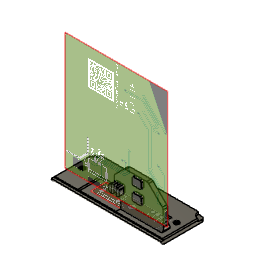
P3_LTE (Autodesk Fusion 360 design; units mm, degrees)
Autodesk Fusion 360 part; units mm, degrees
sketch "草图1" plane through (0, 0, 0) normal (0, 0, 1) x (1, 0, 0)
  line L0 (0, 0) -> (43, 0)
  line L1 (43, 0) -> (43, 17.2)
  line L2 (43, 17.2) -> (0, 17.2)
  line L3 (0, 17.2) -> (0, 0)
  line L4 (0, 17.2) -> (3, 17.2) construction
  line L5 (3, 17.2) -> (3, 9.2) construction
  line L6 (3, 9.2) -> (0, 9.2) construction
  line L7 (0, 9.2) -> (0, 17.2) construction
  line L8 (21.5, 17.2) -> (21.5, 0) construction
  circle A0 centre (3, 9.2) radius 1.025
  circle A1 centre (3, 9.2) radius 2.05
  circle A2 centre (40, 9.2) radius 1.025
  circle A3 centre (40, 9.2) radius 2.05
  dimension "d1" = 43
  dimension "d2" = 17.2
  dimension "d17" = 3
  dimension "d18" = 8
  dimension "d19" = 2.05
  dimension "d20" = 4.1
  constraint horizontal L0
  constraint vertical L1
  constraint horizontal L2
  constraint vertical L3
  constraint coincident L0.start L3.end
  constraint horizontal L4
  constraint vertical L5
  constraint horizontal L6
  constraint vertical L7
  constraint midpoint L2 L8.start
  constraint midpoint L0 L8.end
  constraint coincident L5.end L6.start
  constraint concentric A0 A1
  constraint symmetric L8 A0 A2
  constraint symmetric L8 A1 A3
  measures "d1" distance of L0.start L0.end
  measures "d2" distance of L0.start L2.end
  measures "d17" distance of L2.end L4.end
  measures "d18" distance of L2.end L6.end
  measures "d19" diameter of A0
  measures "d20" diameter of A1
extrude "拉伸1" add sketch "草图1" along normal blind 1.8 contours L0 L1 L2 L3 | A0 | A1 | A2 | A3
sketch "草图2" plane through (0, 0, 1.8) normal (0, 0, 1) x (-1, 0, 0)
  line L0 (0, -17.2) -> (0, 0)
  line L1 (0, 0) -> (-43, 0)
  line L2 (-43, 0) -> (-43, -17.2)
  line L3 (-43, -17.2) -> (0, -17.2)
  circle A0 centre (0, -17.2) radius 2.5
  circle A1 centre (-43, -17.2) radius 2.5
  line L4 (0, 0) -> (-43, 0)
  line L5 (-43, 0) -> (-43, -1)
  line L6 (-43, -1) -> (0, -1)
  line L7 (0, -1) -> (0, 0)
  dimension "d5" = 5
  dimension "d6" = 5
  dimension "d11" = 1
  constraint coincident L0.start L3.end
  constraint coincident L2.end L3.start
  constraint horizontal L4
  constraint vertical L5
  constraint horizontal L6
  constraint vertical L7
  constraint coincident L0.end L1.start
  measures "d5" diameter of A0
  measures "d6" diameter of A1
  measures "d11" distance of L0.end L6.end
extrude "拉伸2" cut sketch "草图2" against normal blind 0.9 contours L0 L3 A0 | L2 L3 A1 picked at (-1.3308, -16.2037) picked at (-41.5409, -16.4033)
fillet "圆角1" radius 1 2 edges at (43, 17.2, 0.45) (0, 17.2, 0.45)
extrude "拉伸3" cut sketch "草图2" against normal blind 0.4 contours L0 L1 L2 L4 L5 L6 L7
fillet "圆角3" radius 1.5 1 edges at (21.5, 0, 0)
chamfer "倒角1" distance 0.4 angle 45 2 edges at (43, 7.85, 1.8) (0, 7.85, 1.8)
extrude "拉伸4" cut sketch "草图1" along normal up to surface (1.8 mm away) contours A0 | A2
extrude "拉伸5" cut sketch "草图1" along normal blind 0.5 contours A1 | A3
chamfer "倒角3" distance 1 angle 45 2 edges at (39.0444, 9.5707, 0.5) (2.0444, 9.5707, 0.5)
chamfer "倒角4" distance 0.2 angle 45 2 edges at (1.0887, 8.4587, 0) (38.0887, 8.4587, 0)
sketch "草图10" plane through (0, 0, 1.8) normal (0, 0, 1) x (-1, 0, 0)
  circle A0 centre (-40, -9.2) radius 1.025
  circle A1 centre (-3, -9.2) radius 1.025
  line L0 (-0.4, -14.7322) -> (-0.4, -1)
  line L1 (-0.4, -1) -> (-42.6, -1)
  line L2 (-42.6, -1) -> (-42.6, -14.7322)
  arc A2 (-40.5, -17.2) -> (-42.6, -14.7322) centre (-43, -17.2) ccw
  line L3 (-40.5, -17.2) -> (-2.5, -17.2)
  arc A3 (-0.4, -14.7322) -> (-2.5, -17.2) centre (0, -17.2) ccw
  line L4 (-40, -9.2) -> (-37.3, -9.2) construction
  line L5 (-37.3, -10) -> (-9.3, -10)
  line L6 (-9.3, -10) -> (-9.3, -3.9)
  line L7 (-9.3, -3.9) -> (-37.3, -3.9)
  line L8 (-37.3, -3.9) -> (-37.3, -10)
  line L9 (-37.3, -9.2) -> (-37.3, -10) construction
  line L10 (-4, -16) -> (-39, -16) construction
  line L11 (-39, -16) -> (-39, -10) construction
  line L12 (-39, -10) -> (-4, -10)
  line L13 (-4, -10) -> (-4, -16) construction
  line L14 (-21.5, -16) -> (-21.5, -10) construction
  line L15 (-21.5, -17.2) -> (-21.5, -1) construction
  line L16 (-37.3, -10) -> (-25.1, -10) construction
  line L17 (-25.1, -10) -> (-25.1, -6.6) construction
  line L18 (-25.1, -6.6) -> (-37.3, -6.6) construction
  line L19 (-37.3, -6.6) -> (-37.3, -10) construction
  circle A4 centre (-25.1, -6.6) radius 0.9
  line L20 (-9.3, -3.9) -> (-24.3, -3.9)
  line L21 (-24.3, -3.9) -> (-24.3, -1.9)
  line L22 (-24.3, -1.9) -> (-9.3, -1.9)
  line L23 (-9.3, -1.9) -> (-9.3, -3.9)
  line L24 (0, -14.7) -> (0, -1)
  line L25 (-43, -1) -> (-43, -14.7)
  line L26 (0, -1) -> (-43, -1) construction
  line L27 (-43, -1) -> (-43, -2.4) construction
  line L28 (-43, -2.4) -> (0, -2.4) construction
  line L29 (0, -2.4) -> (0, -1) construction
  line L30 (0, -2.4) -> (-2.8, -2.4) construction
  line L31 (-43, -2.4) -> (-40.2, -2.4) construction
  line L32 (-2.8, -2.4) -> (-40.2, -2.4)
  line L33 (-40.2, -2.4) -> (-40.2, -3.8)
  line L34 (-40.2, -3.8) -> (-2.8, -3.8)
  line L35 (-2.8, -3.8) -> (-2.8, -2.4)
  line L36 (0, -1) -> (-2.4, -1) construction
  line L37 (-2.4, -1) -> (-2.4, -5.5) construction
  line L38 (-2.4, -5.5) -> (0, -5.5) construction
  line L39 (0, -5.5) -> (0, -1) construction
  line L40 (-43, -1) -> (-40.6, -1) construction
  line L41 (-40.6, -1) -> (-40.6, -5.5) construction
  line L42 (-40.6, -5.5) -> (-43, -5.5) construction
  line L43 (-43, -5.5) -> (-43, -1) construction
  line L44 (-2.4, -5.5) -> (-40.6, -5.5)
  line L45 (-40.6, -5.5) -> (-40.6, -1)
  line L46 (-40.6, -1) -> (-2.4, -1)
  line L47 (-2.4, -1) -> (-2.4, -5.5)
  line L48 (-2.4, -3.8) -> (-2.8, -3.8)
  line L49 (-2.4, -2.4) -> (-2.8, -2.4)
  line L50 (-40.2, -3.8) -> (-40.6, -3.8)
  line L51 (-40.6, -2.4) -> (-40.2, -2.4)
  line L52 (-37.3, -3.9) -> (-37.3, -3.8)
  dimension "d180" = 2.7
  dimension "d181" = 28
  dimension "d182" = 6.1
  dimension "d183" = 0.8
  dimension "d184" = 35
  dimension "d185" = 6
  dimension "d186" = 12.2
  dimension "d187" = 3.4
  dimension "d188" = 1.8
  dimension "d189" = 15
  dimension "d190" = 2
  dimension "d204" = 1.4
  dimension "d205" = 2.8
  dimension "d206" = 2.8
  dimension "d207" = 1.4
  dimension "d210" = 2.4
  dimension "d211" = 4.5
  dimension "d212" = 2.4
  dimension "d213" = 4.5
  constraint coincident A0.centre L4.start
  constraint horizontal L4
  constraint horizontal L5
  constraint vertical L6
  constraint horizontal L7
  constraint vertical L8
  constraint coincident L4.end L8
  constraint perpendicular L4 L9
  constraint horizontal L10
  constraint vertical L11
  constraint horizontal L12
  constraint vertical L13
  constraint collinear L5 L12
  constraint midpoint L10 L14.start
  constraint midpoint L12 L14.end
  constraint midpoint L3 L15.start
  constraint midpoint L1 L15.end
  constraint collinear L14 L15
  constraint horizontal L16
  constraint vertical L17
  constraint horizontal L18
  constraint vertical L19
  constraint coincident L17.end L18.start
  constraint horizontal L20
  constraint vertical L21
  constraint horizontal L22
  constraint vertical L23
  constraint horizontal L26
  constraint vertical L27
  constraint horizontal L28
  constraint vertical L29
  constraint coincident L24.end L26.start
  constraint perpendicular L24 L30
  constraint perpendicular L2 L31
  constraint horizontal L32
  constraint vertical L33
  constraint horizontal L34
  constraint vertical L35
  constraint horizontal L36
  constraint vertical L37
  constraint horizontal L38
  constraint vertical L39
  constraint horizontal L40
  constraint vertical L41
  constraint horizontal L42
  constraint vertical L43
  constraint coincident L25.start L26.end
  constraint horizontal L44
  constraint vertical L45
  constraint horizontal L46
  constraint vertical L47
  constraint coincident L47 L48.start
  constraint perpendicular L35 L48
  constraint coincident L30 L49.start
  constraint coincident L37 L49.start
  constraint coincident L45 L50.end
  constraint perpendicular L45 L50
  constraint coincident L45 L51.start
  constraint coincident L31 L51.start
  constraint coincident L34 L52.end
  constraint perpendicular L34 L52
  measures "d180" distance of A0.centre L4.end
  measures "d181" distance of L5.start L5.end
  measures "d182" distance of L5.start L7.end
  measures "d183" distance of L4.end L5.start
  measures "d184" distance of L10.start L10.end
  measures "d185" distance of L10.start L12.end
  measures "d186" distance of L5.start L16.end
  measures "d187" distance of L5.start L18.end
  measures "d188" diameter of A4
  measures "d189" distance of L6.end L20.end
  measures "d190" distance of L6.end L22.end
  measures "d204" distance of L24.end L28.end
  measures "d205" distance of L28.end L30.end
  measures "d206" distance of L27.end L31.end
  measures "d207" distance of L30.end L34.end
  measures "d210" distance of L24.end L36.end
  measures "d211" distance of L24.end L38.end
  measures "d212" distance of L25.start L40.end
  measures "d213" distance of L25.start L42.end
extrude "拉伸25" cut sketch "草图10" against normal blind 0.8 contours L21 L22 L23 L32 | L21 L23 L32 L34 | L7 L20 L21 L23 L34
extrude "拉伸24" cut sketch "草图10" against normal blind 0.8 contours L6 L7 L8 L20 L44 | L5 L6 L8 L12 L44
chamfer "倒角12" distance 0.8 angle 45 1 edges at (16.8, 1.9, 1.8)
sketch "草图12" plane through (0, 0, 1.8) normal (0, 0, 1) x (-1, 0, 0)
  line L0 (-9.3, -1.1) -> (-9.3, -10)
  line L1 (-9.3, -10) -> (-37.3, -10)
  line L2 (-37.3, -10) -> (-37.3, -3.9)
  line L3 (-37.3, -3.9) -> (-24.3, -3.9)
  line L4 (-24.3, -3.9) -> (-24.3, -1.1)
  line L5 (-24.3, -1.1) -> (-9.3, -1.1)
  line L6 (-0.4, -14.7322) -> (-0.4, -1)
  line L7 (-0.4, -1) -> (-42.6, -1)
  line L8 (-42.6, -1) -> (-42.6, -14.7322)
  arc A0 (-40.5, -17.2) -> (-42.6, -14.7322) centre (-43, -17.2) ccw
  line L9 (-40.5, -17.2) -> (-2.5, -17.2)
  arc A1 (-0.4, -14.7322) -> (-2.5, -17.2) centre (0, -17.2) ccw
  circle A2 centre (-3, -9.2) radius 1.025
  circle A3 centre (-40, -9.2) radius 1.025
  line L10 (-40.6, -1) -> (-2.4, -1)
  line L11 (-2.4, -1) -> (-2.4, -5.5)
  line L12 (-40.6, -5.5) -> (-40.6, -1)
  line L13 (-2.4, -5.5) -> (-40.6, -5.5)
  line L14 (-40.2, -3.8) -> (-2.8, -3.8)
  line L15 (-2.4, -3.8) -> (-2.8, -3.8)
  line L16 (-2.8, -3.8) -> (-2.8, -2.4)
  line L17 (-40.2, -3.8) -> (-40.6, -3.8)
  line L18 (-40.2, -2.4) -> (-40.2, -3.8)
  line L19 (-43, -2.4) -> (0, -2.4)
  line L20 (-9.3, -1.1) -> (-24.3, -1.1)
  line L21 (-9.3, -1.1) -> (-9.3, -10)
  line L22 (-37.3, -6.6) -> (-37.3, -10)
  line L23 (-37.3, -3.9) -> (-37.3, -10)
  line L24 (-39, -10) -> (-4, -10)
  circle A4 centre (-25.1, -6.6) radius 0.9
  circle A5 centre (-25.1, -6.6) radius 0.9
  line L25 (-9.3, -1.9) -> (-24.3, -1.9)
  line L26 (-24.3, -1.9) -> (-24.3, -3.9)
  line L27 (-24.3, -3.9) -> (-37.3, -3.9)
  line L28 (-37.3, -3.9) -> (-37.3, -10)
  line L29 (-37.3, -10) -> (-9.3, -10)
  line L30 (-9.3, -10) -> (-9.3, -1.9)
  line L31 (-24.3, -1.1) -> (-24.3, -1.9)
  line L32 (-24.3, -1.9) -> (-9.3, -1.9)
  line L33 (-9.3, -1.9) -> (-9.3, -1.1)
  line L34 (-9.3, -1.1) -> (-24.3, -1.1)
  line L35 (-37.3, -3.9) -> (-37.3, -3.8)
extrude "拉伸27" add sketch "草图12" along normal blind 2 contours L0 L11 L13 L14 L15 L21 L30 | L2 L12 L13 L14 L17 L23 L28 L35
sketch "草图13" plane through (9.3, 0, 0) normal (1, 0, 0) x (0, 1, 0)
  line L0 (3.8, 1.8) -> (1.1, 1.8)
  line L1 (1.1, 1.8) -> (1.9, 1)
  line L2 (1.9, 1) -> (10, 1)
  line L3 (10, 1) -> (10, 1.8)
  line L4 (10, 1.8) -> (5.5, 1.8)
  line L5 (5.5, 1.8) -> (5.5, 3.8)
  line L6 (5.5, 3.8) -> (3.8, 3.8)
  line L7 (3.8, 3.8) -> (3.8, 1.8)
  line L8 (3.8, 3.8) -> (5.5, 3.8)
  line L9 (5.5, 3.8) -> (5.5, 1.8)
  line L10 (5.5, 1.8) -> (3.8, 1.8)
  line L11 (3.8, 1.8) -> (3.8, 3.8)
  constraint horizontal L8
  constraint vertical L9
  constraint horizontal L10
  constraint vertical L11
  constraint coincident L4.end L5.start
  constraint coincident L6.end L7.start
extrude "拉伸28" add sketch "草图13" along normal up to surface (28 mm away) contours L5 L6 L7 L8 L9 L10 L11
sketch "草图14" plane through (0, 0, 3.8) normal (0, 0, 1) x (-1, 0, 0)
  line L0 (-40.6, -5.5) -> (-2.4, -5.5)
  line L1 (-2.4, -3.8) -> (-40.6, -3.8)
  line L2 (-20.4484, -5.5) -> (-40.6, -5.5)
  line L3 (-40.6, -5.5) -> (-40.6, -3.8)
  line L4 (-40.6, -3.8) -> (-20.4484, -3.8)
  line L5 (-20.4484, -3.8) -> (-20.4484, -5.5)
  line L6 (-2.4, -5.5) -> (-2.4, -3.8)
  line L7 (-40.6, -3.8) -> (-40.6, -5.5)
  constraint horizontal L2
  constraint vertical L3
  constraint horizontal L4
  constraint vertical L5
  constraint coincident L1.end L3.end
  constraint coincident L0 L2.start
extrude "拉伸29" add sketch "草图14" along normal blind 11 contours L0 L1 L2 L3 L4 L5 L7
chamfer "倒角14" distance 7 angle 45 1 edges at (40.6, 4.65, 14.8)
chamfer "倒角14" distance 4 angle 45 1 edges at (20.4484, 4.65, 14.8)
sketch "草图16" plane through (0, 3.8, 0) normal (0, -1, 0) x (1, 0, 0)
  line L0 (24.4484, 14.8) -> (20.4484, 10.8)
  line L1 (20.4484, 10.8) -> (20.4484, 3.8)
  line L2 (20.4484, 3.8) -> (2.4, 3.8)
  line L3 (2.4, 3.8) -> (2.4, 1.8)
  line L4 (2.4, 1.8) -> (9.3, 1.8)
  line L5 (40.6, 1.8) -> (40.6, 7.8)
  line L6 (40.6, 7.8) -> (33.6, 14.8)
  line L7 (33.6, 14.8) -> (24.4484, 14.8)
  line L8 (21.0106, 9.3109) -> (24.5661, 9.3109)
  line L9 (24.5661, 9.3109) -> (24.5661, 6.3199)
  line L10 (24.5661, 6.3199) -> (21.0106, 6.3199)
  line L11 (21.0106, 6.3199) -> (21.0106, 9.3109)
  line L12 (28.3992, 14.78) -> (32.0076, 14.78)
  line L13 (32.0076, 14.78) -> (32.0076, 11.7789)
  line L14 (32.0076, 11.7789) -> (28.3992, 11.7789)
  line L15 (28.3992, 11.7789) -> (28.3992, 14.78)
  line L16 (28.3992, 9.3109) -> (32.0076, 9.3109)
  line L17 (32.0076, 9.3109) -> (32.0076, 6.3199)
  line L18 (32.0076, 6.3199) -> (28.3992, 6.3199)
  line L19 (28.3992, 6.3199) -> (28.3992, 9.3109)
  line L20 (9.3, 1.8) -> (24.3, 1.8)
  line L21 (24.3, 1.8) -> (40.6, 1.8)
  constraint horizontal L8
  constraint vertical L9
  constraint horizontal L10
  constraint vertical L11
  constraint horizontal L12
  constraint vertical L13
  constraint horizontal L14
  constraint vertical L15
  constraint horizontal L16
  constraint vertical L17
  constraint horizontal L18
  constraint vertical L19
  constraint collinear L10 L18
  constraint collinear L8 L16
  constraint collinear L13 L17
  constraint collinear L15 L19
extrude "拉伸30" add sketch "草图16" along normal blind 0.5 contours L12 L13 L14 L15 | L16 L17 L18 L19
extrude "拉伸31" add sketch "草图16" along normal blind 2 contours L8 L9 L10 L11
fillet "圆角10" radius 0.5 12 edges at (28.3992, 3.55, 14.78) (28.3992, 3.55, 11.7789) (32.0076, 3.55, 11.7789) (28.3992, 3.55, 9.3109) (28.3992, 3.55, 6.3199) (32.0076, 3.55, 6.3199) (24.5661, 2.8, 6.3199) (21.0106, 2.8, 6.3199) (21.0106, 2.8, 9.3109) (32.0076, 3.55, 14.78) (32.0076, 3.55, 9.3109) (24.5661, 2.8, 9.3109)
extrude "拉伸32" cut 1 faces at (14.4322, 4.9333, 3.8) along direction (0, 0, -1) up to surface (2 mm away)
chamfer "倒角15" distance 4 angle 45 1 edges at (20.4484, 4.65, 1.8)
chamfer "倒角16" distance 1.5 angle 45 1 edges at (30.8742, 5.5, 1.8)
chamfer "倒角16" distance 1 angle 45 1 edges at (32.45, 3.8, 1.8)
extrude "拉伸33" cut 2 faces at (14.2667, 6.1667, 1) (19.3, 1.9, 1.0001) along direction (0, 0, 1) blind 1
fillet "圆角13" radius 15 1 edges at (30.7742, 4.2, 2)
sketch "草图17" plane through (40.6, 0, 0) normal (1, 0, 0) x (0, 1, 0)
  line L0 (5.5, 7.8) -> (3.8, 7.8)
  line L1 (3.8, 7.8) -> (3.8, 2.8)
  line L2 (3.8, 2.8) -> (2.8, 1.8)
  line L3 (2.8, 1.8) -> (5.5, 1.8)
  line L4 (5.5, 1.8) -> (5.5, 7.8)
  line L5 (3.8, 2.8) -> (5.5, 2.8)
  line L6 (5.5, 2.8) -> (5.5, 12.5)
  line L7 (5.5, 12.5) -> (3.8, 12.5)
  line L8 (3.8, 12.5) -> (3.8, 2.8)
  constraint horizontal L5
  constraint vertical L6
  constraint horizontal L7
  constraint vertical L8
  constraint coincident L1.end L2.start
extrude "拉伸34" cut sketch "草图17" against normal blind 1 contours L0 L1 L4 L5 L6 L8 | L0 L6 L7 L8
fillet "圆角12" radius 1 7 edges at (24.4484, 4.65, 14.8) (20.4484, 4.65, 10.8) (33.6, 4.65, 14.8) (20.4484, 4.65, 5.8) (39.6, 4.65, 8.8) (40.6, 4.65, 2.8) (39.6, 4.65, 2.8)
extrude "拉伸35" cut 2 faces at (31.5186, 3.8, 3.9733) (39.8145, 3.8, 2.9793) along direction (0, 1, 0) blind 0.5
extrude "拉伸36" add 2 faces at (31.1447, 5.5, 7.1333) (39.8145, 5.5, 2.9793) along direction (0, 1, 0) blind 0.5
chamfer "倒角17" distance 0.5 angle 45 1 edges at (30.1242, 6, 3.3)
chamfer "倒角17" distance 0.5 angle 45 1 edges at (31.8648, 4.3, 2.8)
sketch "草图18" plane through (24.5661, 0, 0) normal (1, 0, 0) x (0, 1, 0)
  line L0 (4.3, 8.8109) -> (1.8, 8.8109)
  line L1 (1.8, 8.8109) -> (1.8, 6.8199)
  line L2 (1.8, 6.8199) -> (4.3, 6.8199)
  line L3 (4.3, 6.8199) -> (4.3, 8.8109)
  line L4 (4.3, 8.8109) -> (3.5, 8.8109) construction
  line L5 (3.5, 8.8109) -> (3.5, 6.8199) construction
  line L6 (3.5, 6.8199) -> (4.3, 6.8199) construction
  line L7 (4.3, 6.8199) -> (4.3, 8.8109) construction
  line L8 (3.5, 8.8109) -> (1.8, 8.8109)
  line L9 (1.8, 8.8109) -> (1.8, 6.8199)
  line L10 (1.8, 6.8199) -> (3.5, 6.8199)
  line L11 (3.5, 6.8199) -> (3.5, 8.8109)
  dimension "d255" = 0.8
  constraint horizontal L4
  constraint vertical L5
  constraint horizontal L6
  constraint vertical L7
  constraint coincident L2 L5.end
  constraint coincident L0.start L3.end
  constraint horizontal L8
  constraint vertical L9
  constraint horizontal L10
  constraint vertical L11
  constraint coincident L1.end L2.start
  measures "d255" distance of L0.start L4.end
extrude "拉伸37" add sketch "草图18" along normal blind 0.3 contours L0 L1 L2 L8 L9 L10 L11
sketch "草图19" plane through (0, 1.8, 0) normal (0, -1, 0) x (1, 0, 0)
  arc A0 (24.5661, 8.8109) -> (24.0661, 9.3109) centre (24.0661, 8.8109) ccw
  line L0 (24.0661, 9.3109) -> (21.5106, 9.3109)
  arc A1 (21.5106, 9.3109) -> (21.0106, 8.8109) centre (21.5106, 8.8109) ccw
  line L1 (21.0106, 8.8109) -> (21.0106, 6.8199)
  arc A2 (21.0106, 6.8199) -> (21.5106, 6.3199) centre (21.5106, 6.8199) ccw
  line L2 (21.5106, 6.3199) -> (24.0661, 6.3199)
  arc A3 (24.0661, 6.3199) -> (24.5661, 6.8199) centre (24.0661, 6.8199) ccw
  line L3 (22.7884, 9.3109) -> (22.7884, 6.3199) construction
  line L4 (22.2884, 9.3109) -> (23.2884, 9.3109)
  line L5 (23.2884, 9.3109) -> (23.2884, 6.3199)
  line L6 (23.2884, 6.3199) -> (22.2884, 6.3199)
  line L7 (22.2884, 6.3199) -> (22.2884, 9.3109)
  line L8 (24.5661, 6.8199) -> (24.8661, 6.8199)
  line L9 (24.8661, 6.8199) -> (24.8661, 8.8109)
  line L10 (24.8661, 8.8109) -> (24.5661, 8.8109)
  dimension "d259" = 1
  constraint midpoint L0 L3.start
  constraint midpoint L2 L3.end
  constraint horizontal L4
  constraint vertical L5
  constraint horizontal L6
  constraint vertical L7
  constraint coincident L2 L5.end
  constraint coincident L0 L4.start
  constraint midpoint L3.start L4
  measures "d259" distance of L4.start L4.end
extrude "拉伸38" cut sketch "草图19" against normal blind 2.5 contours L0 L2 L4 L5 L6 L7
sketch "草图20" plane through (21.0106, 0, 0) normal (-1, 0, 0) x (0, -1, 0)
  line L0 (-1.8, 8.8109) -> (-4.3, 8.8109)
  line L1 (-4.3, 8.8109) -> (-4.3, 6.8199)
  line L2 (-4.3, 6.8199) -> (-1.8, 6.8199)
  line L3 (-1.8, 6.8199) -> (-1.8, 8.8109)
  line L4 (-4.3, 8.8109) -> (-3.5, 8.8109) construction
  line L5 (-3.5, 8.8109) -> (-3.5, 6.8199) construction
  line L6 (-3.5, 6.8199) -> (-4.3, 6.8199) construction
  line L7 (-4.3, 6.8199) -> (-4.3, 8.8109) construction
  line L8 (-3.5, 8.8109) -> (-1.8, 8.8109)
  line L9 (-1.8, 8.8109) -> (-1.8, 6.8199)
  line L10 (-1.8, 6.8199) -> (-3.5, 6.8199)
  line L11 (-3.5, 6.8199) -> (-3.5, 8.8109)
  dimension "d262" = 0.8
  constraint horizontal L4
  constraint vertical L5
  constraint horizontal L6
  constraint vertical L7
  constraint coincident L2 L5.end
  constraint coincident L0.end L1.start
  constraint horizontal L8
  constraint vertical L9
  constraint horizontal L10
  constraint vertical L11
  constraint coincident L2.end L3.start
  measures "d262" distance of L0.end L4.end
extrude "拉伸39" add sketch "草图20" along normal blind 0.3 contours L0 L2 L3 L8 L9 L10 L11
fillet "圆角15" radius 0.5 4 edges at (22.2884, 4.3, 7.8154) (23.2884, 4.3, 7.8154) (22.2884, 1.8, 7.8154) (23.2884, 1.8, 7.8154)
named bodies: "P3_LTE"
